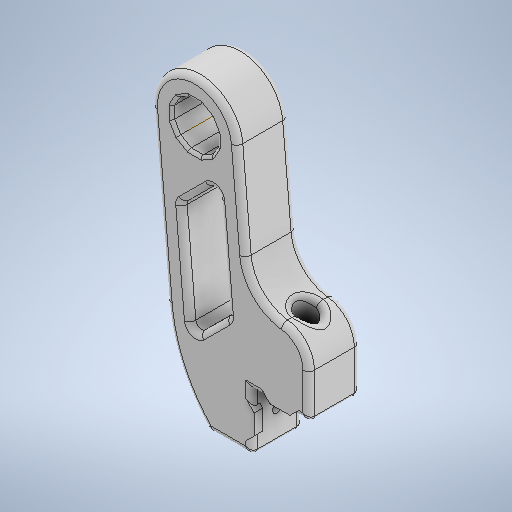
# Autodesk Inventor part: Z-Endstop
Saved by Autodesk Inventor 2025.3 (Build 293356030, 356C)
## iProperties
Created: 2025-10-01
Part Number: Z-Endstop
Material: Generic
Document SubType Name: Modeling
Designer: tvoko
Density: 1 g/cm^3
Appearance: Default
Author: tvoko
Autodesk Inventor part; units mm, degrees
ref_plane "YZ Plane" through (0, 0, 0) normal (1, 0, 0) x (0, 1, 0)
ref_plane "XZ Plane" through (0, 0, 0) normal (0, 1, 0) x (-1, 0, 0)
ref_plane "XY Plane" through (0, 0, 0) normal (0, 0, 1) x (1, 0, 0)
sketch "Sketch1" plane through (0, 0, 0) normal (0, 0, 1) x (1, 0, 0)
  line L0 (-10.05, 10.05) -> (10.05, 10.05)
  line L1 (10.05, 10.05) -> (10.05, -10.05)
  line L2 (10.05, -10.05) -> (-10.05, -10.05)
  line L3 (-10.05, -10.05) -> (-10.05, 10.05)
  line L4 (0, 10.05) -> (0, -10.05) construction
  line L5 (-10.05, 0) -> (10.05, 0) construction
  line L6 (-10.05, 4.5) -> (-9.05, 3.5)
  line L7 (-9.05, 3.5) -> (-9.05, -3.5)
  line L8 (-9.05, -3.5) -> (-10.05, -4.5)
  line L9 (-4.5, 10.05) -> (-3.5, 9.05)
  line L10 (-3.5, 9.05) -> (3.5, 9.05)
  line L11 (3.5, 9.05) -> (4.5, 10.05)
  line L12 (10.05, 10.05) -> (10.05, 25.05)
  line L13 (-10.05, -10.05) -> (-25.05, -10.05)
  line L14 (-25.05, -10.05) -> (-25.05, 10.05)
  line L15 (-9.95, 25.05) -> (-25.05, 10.05)
  line L16 (10.05, 25.05) -> (-9.95, 25.05)
  line L17 (-9.95, 25.05) -> (-9.95, 10.05)
  line L18 (-10.05, 9.95) -> (-25.05, 9.95)
  circle A0 centre (-30, 80) radius 7.95 construction
  arc A1 (-15.0614, 81.3561) -> (-44.9386, 78.6439) centre (-30, 80) ccw
  line L19 (-15.0614, 81.3561) -> (-12.1198, 48.9517)
  line L20 (-44.9386, 78.6439) -> (-39.8271, 22.3378)
  line L21 (-39.8271, 22.3378) -> (-25.05, -10.05) construction
  line L22 (-9.95, 25.05) -> (-39.8271, 22.3378) construction
  arc A2 (-39.8271, 22.3378) -> (-25.05, -10.05) centre (13.7055, 27.1974) ccw
  line L23 (-9.95, 25.05) -> (0.7163, 35.6457) construction
  arc A3 (10.05, 25.05) -> (0.7163, 35.6457) centre (-0.631, 25.05) ccw
  arc A4 (-12.1198, 48.9517) -> (0.7163, 35.6457) centre (2.5779, 50.286) ccw
  line L24 (-12.1198, 48.9517) -> (-9.95, 25.05) construction
  line L25 (-25.4101, 87.95) -> (-20.8201, 80)
  line L26 (-20.8201, 80) -> (-25.4101, 72.05)
  line L27 (-25.4101, 72.05) -> (-34.5899, 72.05)
  line L28 (-34.5899, 72.05) -> (-39.1799, 80)
  line L29 (-39.1799, 80) -> (-34.5899, 87.95)
  line L30 (-34.5899, 87.95) -> (-25.4101, 87.95)
  line L31 (-30, 89.1799) -> (-22.05, 84.5899)
  line L32 (-22.05, 84.5899) -> (-22.05, 75.4101)
  line L33 (-22.05, 75.4101) -> (-30, 70.8201)
  line L34 (-30, 70.8201) -> (-37.95, 75.4101)
  line L35 (-37.95, 75.4101) -> (-37.95, 84.5899)
  line L36 (-37.95, 84.5899) -> (-30, 89.1799)
  line L37 (-24.7954, 63.8653) -> (-34.006, 54.7158)
  line L38 (-34.5883, 53.1161) -> (-31.5366, 19.4995)
  line L39 (-28.1353, 18.2615) -> (-18.9247, 27.411)
  line L40 (-18.3424, 29.0107) -> (-21.3941, 62.6272)
  arc A5 (-21.3941, 62.6272) -> (-24.7954, 63.8653) centre (-23.3859, 62.4464) ccw
  arc A6 (-18.9247, 27.411) -> (-18.3424, 29.0107) centre (-20.3343, 28.8299) ccw
  arc A7 (-31.5366, 19.4995) -> (-28.1353, 18.2615) centre (-29.5448, 19.6804) ccw
  arc A8 (-34.006, 54.7158) -> (-34.5883, 53.1161) centre (-32.5965, 53.2969) ccw
  point P0 (0, 0)
  point P1 (0, 0)
  point P2 (0, 9.05)
  point P3 (-9.05, 0)
  point P4 (-30, 87.95)
  point P5 (-33.975, 86.8849)
  point P6 (-22.05, 82.1302)
  point P7 (-22.05, 77.8698)
  point P8 (-24.1802, 74.1802)
  point P9 (-27.8698, 72.05)
  point P10 (-32.1302, 72.05)
  point P11 (-35.8198, 74.1802)
  point P12 (-37.95, 77.8698)
  point P13 (-37.95, 82.1302)
  point P14 (-27.8698, 87.95)
  point P15 (-24.1802, 85.8198)
  point P16 (-35.8198, 85.8198)
  point P17 (-32.1302, 87.95)
  dimension "d0" = 20.1
  dimension "d1" = 7
  dimension "d2" = 1
  dimension "d3" = 135
  dimension "d4" = 1
  dimension "d5" = 7
  dimension "d6" = 135
  dimension "d8" = 15
  dimension "d9" = 15
  dimension "d18" = 20
  dimension "d19" = 20
  dimension "d61" = 30
  dimension "d62" = 80
  dimension "d63" = 15.9
  dimension "d64" = 30
  dimension "d65" = 24
  dimension "d72" = 2
  dimension "d73" = 8
  dimension "d75" = 8
  dimension "d76" = 8
  dimension "d77" = 30
  constraints: 82 end point, 18 point on circle, 14 tangent, 9 centre point, 9 midpoint, 9 point on line, 7 parallel, 7 perpendicular, 5 horizontal, 4 coincident, 4 equal length, 3 equal radius, 2 vertical, 1 collinear, 26 other
  measures "d0" distance of L0.start L0.end
  measures "d1" distance of L9.end L10.end
  measures "d2" distance between parallel lines of L0 L10
  measures "d3" angle of L10 L11
  measures "d4" distance between parallel lines of L3 L7
  measures "d5" distance of L6.end L7.end
  measures "d6" angle of L7 L6
  measures "d8" distance of L2.end L13.end
  measures "d9" distance of L0.end L12.end
  measures "d18" distance of L12.end L15.start
  measures "d19" distance between parallel lines of L13 L18
  measures "d61" distance from line of L4 A0.centre
  measures "d62" distance from line of A0.centre L5
  measures "d63" diameter of A0
  measures "d64" diameter of A1
  measures "d65" distance of L19.end L15.start
  measures "d72" radius of A5
  measures "d73" distance between parallel lines of L19 L40
  measures "d75" distance between parallel lines of L20 L38
  measures "d76" distance between parallel lines of L15 L39
  measures "d77" distance between parallel lines of L39 L37
extrude "Extrusion1" add sketch "Sketch1" along normal mid plane 18 contours L3 L18 L14 L15 L17 L0 | L17 L16 L12 L0 | L3 L13 L14 L18 | L0 L11 L10 L9 | L15 L14 A2 L20 A1 L19 A4 A3 L16 | L6 L7 L8 L3 | L25 L31 L30 | L31 L32 L25 | L30 L36 L31 | L25 L26 L32 | L36 L29 L30 | L32 L33 L26 | L29 L35 L36 | L26 L27 L33 | L35 L28 L29 | L33 L34 L27 | L28 L34 L35 | L27 L28 L34
fillet "Fillet1" radius 1 2 edges at (10.05, 10.05, 0) (-10.05, -10.05, 0)
sketch "Sketch2" plane through (-4.5, 9.05, -9) normal (0, -1, 0) x (-1, 0, 0)
  line L0 (-9, -18) -> (-13.55, -18) projected
  line L1 (-9, 0) -> (-9, -18) projected
  line L2 (0, 0) -> (0, -18) projected
  circle A0 centre (-4.5, -9) radius 1.55
  circle A1 centre (-4.5, -9) radius 3.5
  line L3 (5.55, 0) -> (5.55, -18) projected
  line L4 (0, 0) -> (5.55, 0) projected
  line L5 (-8, 0) -> (-1, 0) projected
  line L6 (-13.55, 0) -> (-9, 0) projected
  line L7 (-13.55, -18) -> (-13.55, 0) projected
  line L8 (5.55, -18) -> (0, -18) projected
  line L9 (-9, -9) -> (0, -9) construction
  line L10 (-9, -15) -> (0, -15)
  line L11 (0, -15) -> (0, -3)
  line L12 (0, -3) -> (-9, -3)
  line L13 (-9, -3) -> (-9, -15)
  point P0 (-4.5, -9)
  point P1 (-1, 0)
  point P2 (0, -15)
  dimension "d26" = 3.1
  dimension "d27" = 7
  dimension "d66" = 12
  constraints: 10 end point, 4 midpoint, 2 centre point, 2 coincident, 2 parallel, 2 point on line, 1 horizontal, 1 perpendicular, 1 other
  measures "d26" diameter of A0
  measures "d27" diameter of A1
  measures "d66" distance between parallel lines of L12 L10
extrude "Extrusion3" cut sketch "Sketch2" against normal through all contours A0 | A1
sketch "Sketch3" plane through (-9.05, -4.5, -9) normal (1, 0, 0) x (0, 0, 1)
  line L0 (0, -14.55) -> (0, -9) projected
  line L1 (18, -9) -> (18, -14.55) projected
  line L2 (0, -9) -> (18, -9) projected
  line L3 (0, 0) -> (18, 0) projected
  circle A0 centre (9, -4.5) radius 3.5
  circle A1 centre (9, -4.5) radius 1.55
  line L4 (0, -14.55) -> (18, -14.55) projected
  line L5 (18, 4.55) -> (18, 0) projected
  line L6 (0, -8) -> (0, -1) projected
  line L7 (9, -9) -> (9, 0) construction
  line L8 (0, 4.55) -> (18, 4.55) projected
  line L9 (0, 0) -> (0, 4.55) projected
  line L10 (0, -9) -> (18, -9) projected
  line L11 (0, 0) -> (18, 0) projected
  line L12 (15, -9) -> (3, -9)
  line L13 (3, -9) -> (3, 0)
  line L14 (3, 0) -> (15, 0)
  line L15 (15, 0) -> (15, -9)
  point P0 (9, -4.5)
  point P1 (0, -1)
  point P2 (15, 0)
  point P3 (3, 0)
  point P4 (3, -9)
  dimension "d30" = 7
  dimension "d31" = 3.1
  dimension "d69" = 12
  constraints: 10 end point, 5 midpoint, 2 centre point, 2 coincident, 2 parallel, 2 point on line, 1 horizontal, 1 perpendicular, 1 other
  measures "d30" diameter of A0
  measures "d31" diameter of A1
  measures "d69" distance between parallel lines of L13 L15
extrude "Extrusion4" cut sketch "Sketch3" against normal through all contours A0 | A1
extrude "Extrusion5" add sketch "Sketch2" against normal blind 4 contours A1
extrude "Extrusion6" add sketch "Sketch3" against normal blind 4 contours A0
extrude "Extrusion9" cut sketch "Sketch2" against normal up to surface (1 mm away) contours L1 L12 L2 L10 | A1
extrude "Extrusion10" cut sketch "Sketch3" against normal up to surface (1 mm away) contours L13 L3 L15 L2 | A0
fillet "Fillet5" radius 2 49 edges at (-25.05, -10.05, 0) (-18.4549, 28.1458, -9) (-19.8683, 45.819, -9) (-22.7018, 64.3258, -9) (-29.4007, 59.2906, -9) (-34.4758, 53.981, -9) (-33.0624, 36.3078, -9) (-30.2289, 17.801, -9) (-23.53, 22.8362, -9) (-34.4758, 53.981, 9) (-29.4007, 59.2906, 9) (-22.7018, 64.3258, 9) (-19.8683, 45.819, 9) (-18.4549, 28.1458, 9) (-23.53, 22.8362, 9) (-30.2289, 17.801, 9) (-33.0624, 36.3078, 9) (-8.0435, 40.0396, -9) (7.3838, 32.1102, -9) (10.05, 18.05, -9) (9.7571, 10.3429, -9) (6.775, 10.05, -9) (-31.3561, 94.9386, -9) (-42.3829, 50.4908, -9) (-35.1976, 4.885, -9) (-13.5906, 65.1539, -9) (-31.3561, 94.9386, 9) (-42.3829, 50.4908, 9) (-35.1976, 4.885, 9) (-8.0435, 40.0396, 9) (7.3838, 32.1102, 9) (10.05, 18.05, 9) (9.7571, 10.3429, 9) (6.775, 10.05, 9) (-13.5906, 65.1539, 9) (-7.275, 10.05, -9) (-10.05, 7.275, -9) (-10.3429, -9.7571, -9) (-18.05, -10.05, -9) (-10.05, -6.775, -9) (-10.3429, -9.7571, 9) (-10.05, -6.775, 9) (-18.05, -10.05, 9) (-10.05, 7.275, 9) (-7.275, 10.05, 9) (-2.4381, 36.4064, 2.5111) (-2.4366, 36.4059, -2.5125) (3.5, 34.8998, 0.0001) (-32.5693, -0.1522, -3.4967)
fillet "Fillet6" radius 1 24 edges at (-36.8849, 83.975, -9) (-33.975, 86.8849, -9) (-30, 87.95, -9) (-26.025, 86.8849, -9) (-23.1151, 83.975, -9) (-22.05, 80, -9) (-23.1151, 76.025, -9) (-26.025, 73.1151, -9) (-30, 72.05, -9) (-33.975, 73.1151, -9) (-36.8849, 76.025, -9) (-37.95, 80, -9) (-30, 87.95, 9) (-33.975, 86.8849, 9) (-36.8849, 83.975, 9) (-37.95, 80, 9) (-36.8849, 76.025, 9) (-33.975, 73.1151, 9) (-30, 72.05, 9) (-26.025, 73.1151, 9) (-23.1151, 76.025, 9) (-22.05, 80, 9) (-23.1151, 83.975, 9) (-26.025, 86.8849, 9)
body "Solid1"
